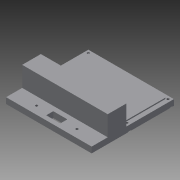
# Autodesk Inventor part: Solonoid holder
Saved by Autodesk Inventor 2015 (Build 190159000, 159)
## iProperties
Created: 2015-11-10
Part Number: Solonoid holder
Material: Generic
Document SubType Name: Modeling
Designer: Lauszus
Density: 1 g/cm^3
Appearance: Default
Author: Lauszus
Autodesk Inventor part; units mm, degrees
ref_plane "YZ Plane" through (0, 0, 0) normal (1, 0, 0) x (0, 1, 0)
ref_plane "XZ Plane" through (0, 0, 0) normal (0, 1, 0) x (-1, 0, 0)
ref_plane "XY Plane" through (0, 0, 0) normal (0, 0, 1) x (1, 0, 0)
sketch "Sketch1" plane through (0, 0, 0) normal (0, 0, 1) x (1, 0, 0)
  line L0 (-36.7256, 32.4279) -> (36.0744, 32.4279)
  line L1 (36.0744, 32.4279) -> (36.0744, -37.5721)
  line L2 (36.0744, -37.5721) -> (-36.7256, -37.5721)
  line L3 (-36.7256, -37.5721) -> (-36.7256, 32.4279)
  point P0 (0, 0)
  dimension "d0" = 72.8
  dimension "d1" = 70
  constraints: 8 end point, 2 parallel, 1 horizontal, 1 perpendicular
  measures "d0" distance of L1.end L2.end
  measures "d1" distance of L0.end L1.end
extrude "Extrusion1" add sketch "Sketch1" along normal blind 5
sketch "Sketch14" plane through (0, 0, 5) normal (0, 0, 1) x (1, 0, 0)
  line L0 (-33.0256, 28.7279) -> (32.3744, 28.7279)
  line L1 (32.3744, 28.7279) -> (32.3744, -4.0721)
  line L2 (32.3744, -4.0721) -> (-33.0256, -4.0721)
  line L3 (-33.0256, -4.0721) -> (-33.0256, 28.7279)
  line L4 (-36.7256, 32.4279) -> (-36.7256, -37.5721) projected
  line L5 (36.0744, -37.5721) -> (36.0744, 32.4279) projected
  line L6 (36.0744, 32.4279) -> (-36.7256, 32.4279) projected
  line L7 (-36.7256, -23.9721) -> (36.0744, -23.9721) projected
  point P0 (0, 0)
  dimension "d92" = 3.7
  dimension "d93" = 3.7
  dimension "d94" = 3.7
  dimension "d99" = 32.8
  constraints: 8 end point, 2 parallel, 1 horizontal, 1 perpendicular
  measures "d92" distance between parallel lines of L4 L3
  measures "d93" distance between parallel lines of L5 L1
  measures "d94" distance between parallel lines of L6 L0
  measures "d99" distance of L2.end L0.start
extrude "Extrusion13" add sketch "Sketch14" along normal blind 1 contours L0 L1 L2 L3
sketch "Sketch15" plane through (0, 0, 0) normal (0, 0, -1) x (-1, 0, 0)
  circle A0 centre (-33.5744, 29.9279) radius 1
  line L0 (36.7256, 32.4279) -> (-36.0744, 32.4279) projected
  line L1 (-36.0744, 32.4279) -> (-36.0744, -37.5721) projected
  line L2 (0.3256, 31.1231) -> (0.3256, 16.9299)
  circle A1 centre (34.2256, 29.9279) radius 1
  line L3 (-36.0744, -7.5721) -> (36.7256, -7.5721)
  line L4 (-36.0744, 12.4279) -> (-22.7568, 12.4279)
  circle A2 centre (-33.5744, -5.0721) radius 1
  circle A3 centre (34.2256, -5.0721) radius 1
  point P0 (0, 0)
  dimension "d100" = 2
  dimension "d101" = 2.5
  dimension "d102" = 2.5
  dimension "d103" = 40
  dimension "d104" = 20
  constraints: 6 end point, 4 centre point, 3 symmetric about line, 2 point on line, 1 horizontal, 1 perpendicular, 1 vertical, 3 other
  measures "d100" diameter of A0
  measures "d101" distance from line of A0.centre L0
  measures "d102" distance from line of A0.centre L1
  measures "d103" distance between parallel lines of L3 L0
  measures "d104" distance between parallel lines of L3 L4
hole "Hole2" at (33.5744, 29.9279, 0) at (-34.2256, 29.9279, 0) at (-34.2256, -5.0721, 0) at (33.5744, -5.0721, 0) direction (0, 0, 1) diameter 2 end through all countersink diameter 6 countersink angle 90
sketch "Sketch18" plane through (0, 0, 5) normal (0, 0, 1) x (1, 0, 0)
  line L0 (-36.7256, -37.5721) -> (-36.7256, -6.7304) projected
  line L1 (36.0744, -37.5721) -> (36.0744, 32.4279) projected
  line L2 (-36.7256, -7.9721) -> (36.0744, -7.9721)
  line L3 (36.0744, -7.9721) -> (36.0744, -23.8721)
  line L4 (36.0744, -23.8721) -> (-36.7256, -23.8721)
  line L5 (-36.7256, -23.8721) -> (-36.7256, -7.9721)
  line L6 (-33.0256, -4.0721) -> (32.3744, -4.0721) projected
  line L7 (-36.7256, -37.5721) -> (36.0744, -37.5721) projected
  point P0 (0, 0)
  dimension "d123" = 3.9
  dimension "d124" = 13.7
  constraints: 8 end point, 2 parallel, 2 point on line, 1 horizontal, 1 perpendicular
  measures "d123" distance between parallel lines of L2 L6
  measures "d124" distance between parallel lines of L7 L4
extrude "Extrusion16" add sketch "Sketch18" along normal blind 17 contours L0 L2 L1 L4
sketch "Sketch19" plane through (0, 0, 5) normal (0, 0, 1) x (1, 0, 0)
  line L0 (-36.7256, -37.5721) -> (36.0744, -37.5721) projected
  line L1 (-0.3256, -37.5721) -> (-0.3256, -23.8721)
  line L2 (-36.7256, -23.8721) -> (36.0744, -23.8721) projected
  circle A0 centre (-17.5256, -30.8221) radius 1
  circle A1 centre (16.8744, -30.8221) radius 1
  point P0 (0, 0)
  dimension "d127" = 2
  dimension "d128" = 2
  dimension "d129" = 6.75
  dimension "d130" = 6.75
  dimension "d131" = 17.2
  dimension "d132" = 17.2
  constraints: 2 centre point, 2 end point, 2 midpoint
  measures "d127" diameter of A0
  measures "d128" diameter of A1
  measures "d129" distance from line of L0 A1.centre
  measures "d130" distance from line of L0 A0.centre
  measures "d131" distance from line of L1 A0.centre
  measures "d132" distance from line of A1.centre L1
extrude "Extrusion17" cut sketch "Sketch19" against normal through all
sketch "Sketch20" plane through (0, 0, 5) normal (0, 0, 1) x (1, 0, 0)
  line L0 (-6.3256, -27.8221) -> (5.6744, -27.8221)
  line L1 (5.6744, -27.8221) -> (5.6744, -33.8221)
  line L2 (5.6744, -33.8221) -> (-6.3256, -33.8221)
  line L3 (-6.3256, -33.8221) -> (-6.3256, -27.8221)
  line L4 (-36.7256, -37.5721) -> (36.0744, -37.5721) projected
  line L5 (-36.7256, -23.8721) -> (-36.7256, -37.5721) projected
  point P0 (0, 0)
  dimension "d135" = 12
  dimension "d136" = 6
  dimension "d137" = 3.75
  dimension "d138" = 30.4
  constraints: 8 end point, 2 parallel, 1 horizontal, 1 perpendicular
  measures "d135" distance of L1.end L2.end
  measures "d136" distance of L0.end L1.end
  measures "d137" distance between parallel lines of L4 L2
  measures "d138" distance between parallel lines of L3 L5
extrude "Extrusion18" cut sketch "Sketch20" against normal through all
body "Solid1"
